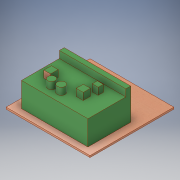
# Autodesk Inventor part: building_1
Saved by Autodesk Inventor 2019 (Build 230136000, 136)
## iProperties
Created: 2020-04-29
Part Number: building_1
Material: Wood (Oak)
Document SubType Name: Modeling
Designer: infinity
Density: 0.76 g/cm^3
Appearance: White Oak - Natural Medium Gloss
Author: infinity
Autodesk Inventor part; units mm, degrees
ref_plane "YZ Plane" through (0, 0, 0) normal (1, 0, 0) x (0, 1, 0)
ref_plane "XZ Plane" through (0, 0, 0) normal (0, 1, 0) x (-1, 0, 0)
ref_plane "XY Plane" through (0, 0, 0) normal (0, 0, 1) x (1, 0, 0)
sketch "Sketch1" plane through (0, 0, 0) normal (0, 1, 0) x (-1, 0, 0)
  line L0 (0, 0) -> (1219.2, 0)
  line L1 (1219.2, 0) -> (1219.2, -1219.2)
  line L2 (1219.2, -1219.2) -> (0, -1219.2)
  line L3 (0, -1219.2) -> (0, 0)
  dimension "d0" = 1219.2
  dimension "d1" = 1219.2
  constraints: 8 end point, 2 parallel, 1 horizontal, 1 perpendicular
  measures "d0" distance of L0.end L1.end
  measures "d1" distance of L1.end L2.end
extrude "Extrusion1" add sketch "Sketch1" along normal blind 25.4
sketch "Sketch2" plane through (0, 25.4, 0) normal (0, 1, 0) x (1, 0, 0)
  line L0 (-1088.9403, 92.3181) -> (-122.6171, 92.3181)
  line L1 (-122.6171, 92.3181) -> (-122.6171, 714.5717)
  line L2 (-122.6171, 714.5717) -> (-1088.9403, 714.5717)
  line L3 (-1088.9403, 714.5717) -> (-1088.9403, 92.3181)
  point P0 (0, 0)
  constraints: 8 end point, 2 parallel, 1 horizontal, 1 perpendicular
extrude "Extrusion2" add sketch "Sketch2" along normal blind 457.2
sketch "Sketch3" plane through (0, 482.6, 0) normal (0, 1, 0) x (1, 0, 0)
  line L0 (-1088.9403, 92.3181) -> (-1088.9403, 714.5717) projected
  line L1 (-122.6171, 92.3181) -> (-122.6171, 714.5717) projected
  line L2 (-1088.9403, 643.7299) -> (-122.6171, 643.7299)
  line L3 (-122.6171, 643.7299) -> (-122.6171, 92.3181)
  line L4 (-122.6171, 92.3181) -> (-1088.9403, 92.3181)
  line L5 (-1088.9403, 92.3181) -> (-1088.9403, 643.7299)
  line L6 (-954.3907, 283.1597) -> (-856.609, 283.1597)
  line L7 (-856.609, 283.1597) -> (-856.609, 393.1642)
  line L8 (-856.609, 393.1642) -> (-954.3907, 393.1642)
  line L9 (-954.3907, 393.1642) -> (-954.3907, 283.1597)
  line L10 (-430.8509, 462.4262) -> (-343.2547, 462.4262)
  line L11 (-343.2547, 462.4262) -> (-343.2547, 537.7997)
  line L12 (-343.2547, 537.7997) -> (-430.8509, 537.7997)
  line L13 (-430.8509, 537.7997) -> (-430.8509, 462.4262)
  circle A0 centre (-791.4211, 232.2317) radius 53.9356
  circle A1 centre (-650.8599, 232.2317) radius 56.421
  line L14 (-489.9274, 288.6527) -> (-387.0528, 288.6527)
  line L15 (-387.0528, 288.6527) -> (-387.0528, 393.1642)
  line L16 (-387.0528, 393.1642) -> (-489.9274, 393.1642)
  line L17 (-489.9274, 393.1642) -> (-489.9274, 288.6527)
  point P0 (0, 0)
  constraints: 32 end point, 8 parallel, 4 horizontal, 4 perpendicular, 2 centre point, 1 point on line
extrude "Extrusion3" cut sketch "Sketch3" against normal blind 101.6
sketch "Sketch4" plane through (-122.6171, 25.4, -714.5717) normal (0, 0, -1) x (-1, 0, 0)
  line L0 (0, 0) -> (966.3232, 0) projected
  line L1 (243.2512, 0) -> (327.8074, 0)
  line L2 (327.8074, 0) -> (327.8074, 181.9254)
  line L3 (327.8074, 181.9254) -> (243.2512, 181.9254)
  line L4 (243.2512, 181.9254) -> (243.2512, 0)
  line L5 (456.2679, 216.0731) -> (763.5973, 216.0731)
  line L6 (763.5973, 216.0731) -> (763.5973, 72.9779)
  line L7 (763.5973, 72.9779) -> (456.2679, 72.9779)
  line L8 (456.2679, 72.9779) -> (456.2679, 216.0731)
  line L9 (26.9824, 216.0731) -> (196.0948, 216.0731)
  line L10 (196.0948, 216.0731) -> (196.0948, 72.9779)
  line L11 (196.0948, 72.9779) -> (26.9824, 72.9779)
  line L12 (26.9824, 72.9779) -> (26.9824, 216.0731)
  point P0 (-122.6171, -25.4)
  constraints: 24 end point, 6 parallel, 3 horizontal, 3 perpendicular, 3 point on line
extrude "Extrusion4" cut sketch "Sketch4" against normal blind 25.4
equation "\"d1\" = d0"
body "Solid1"
